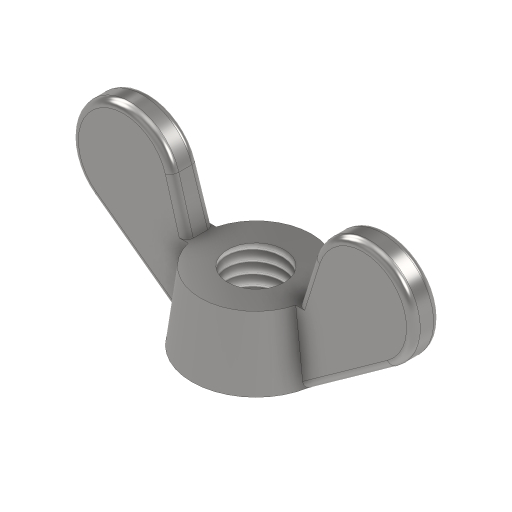
# Autodesk Inventor part: Part38FlyNut
Saved by Autodesk Inventor 2023.2 (Build 272271030, 271C)
## iProperties
Created: 2023-09-07
Part Number: Part38FlyNut
Material: Steel, Carbon
Document SubType Name: Modeling
Designer: User
Density: 7.85 g/cm^3
Appearance: Semi-Polished
Mass: 15.1733 g
Surface Area: 15.3566 cm^2
Volume: 1.9329 cm^3
Author: User
Autodesk Inventor part; units mm, degrees
ref_plane "YZ Plane" through (0, 0, 0) normal (1, 0, 0) x (0, 1, 0)
ref_plane "XZ Plane" through (0, 0, 0) normal (0, 1, 0) x (-1, 0, 0)
ref_plane "XY Plane" through (0, 0, 0) normal (0, 0, 1) x (1, 0, 0)
sketch "Sketch1" plane through (0, 0, 0) normal (1, 0, 0) x (0, 1, 0)
  line L0 (0, 1.75) -> (18, 1.5)
  line L1 (18, 1.5) -> (18, -1.5)
  line L2 (18, -1.5) -> (0, -1.75)
  line L3 (0, -1.75) -> (0, 1.75)
  point P0 (0, 0)
  point P1 (0, 0)
  point P2 (18, 0)
  dimension "d0" = 3.5
  dimension "d1" = 3
  dimension "d2" = 18
  constraints: 8 end point, 2 midpoint, 1 coincident, 1 horizontal alignment, 1 parallel, 1 vertical
  measures "d0" distance of L2.end L0.start
  measures "d1" distance of L0.end L1.end
  measures "d2" distance between parallel lines of L3 L1
extrude "Extrusion1" add sketch "Sketch1" along normal mid plane 40
sketch "Sketch2" plane through (0, 0, 0) normal (0, 0, 1) x (1, 0, 0)
  line L0 (-6.5, 8) -> (6.5, 8)
  line L1 (6.5, 8) -> (7.5, 0)
  line L2 (7.5, 0) -> (-7.5, 0)
  line L3 (-7.5, 0) -> (-6.5, 8)
  arc A0 (17.4822, 7.1138) -> (8.263, 13.7569) centre (14, 12) ccw
  line L4 (-20, 18) -> (20, 18) projected
  line L5 (20, 0) -> (20, 18) projected
  line L6 (8.263, 13.7569) -> (6.5, 8)
  line L7 (17.4822, 7.1138) -> (7.5, 0)
  line L8 (0, -4.0751) -> (0, 24.4507) projected
  arc A1 (-8.263, 13.7569) -> (-17.4822, 7.1138) centre (-14, 12) ccw
  line L9 (-8.263, 13.7569) -> (-6.5, 8)
  line L10 (-17.4822, 7.1138) -> (-7.5, 0)
  point P0 (0, 0)
  point P1 (0, 0)
  dimension "d5" = 8
  dimension "d6" = 15
  dimension "d7" = 13
  dimension "d8" = 6
  constraints: 16 end point, 4 point on circle, 4 tangent, 3 symmetric about line, 2 centre point, 1 coincident, 1 equal length, 1 horizontal, 1 midpoint, 1 parallel, 1 other
  measures "d5" distance between parallel lines of L2 L0
  measures "d6" distance of L1.end L2.end
  measures "d7" distance of L0.start L0.end
  measures "d8" radius of A0
extrude "Extrusion2" cut sketch "Sketch2" along normal mid plane 3.5 contours L0 L8 L2 L3 | L3 L10 A1 L9 | L0 L1 L2 L8 | L6 A0 L7 L1 keep common part
sketch "Sketch3" plane through (0, 0, 0) normal (0, 0, 1) x (1, 0, 0)
  line L0 (6.5, 8) -> (7.5, 0) projected
  line L1 (0, -4.0751) -> (0, 24.4507) projected
  line L2 (0, 8) -> (6.5, 8)
  line L3 (0, 0) -> (7.5, 0)
  constraints: 4 end point, 1 horizontal, 1 perpendicular, 1 point on line
revolve "Revolution1" add sketch "Sketch3" angle 360 about axis through (0, -4.0751, 0) along (0, 1, 0)
sketch "Sketch5" plane through (6.5, 8, 1.6389) normal (0, 1, 0) x (1, 0, 0)
  arc A0 (-0.21, 3.2778) -> (-12.79, 3.2778) centre (-6.5, 1.6389) ccw projected
  point P0 (-6.5, 1.6389)
  constraints: 1 coincident
hole "Hole1" at (0, 8, 0) direction (0, -1, 0) diameter 6.647 end through all thread size "M8x1.25" class "6H" standard "ISO Metric profile"
fillet "Fillet1" radius 0.8 16 edges at (-10.4322, 16.824, 1.5163) (-19.3335, 9.2516, 1.6215) (-7.3815, 10.8784, 1.5989) (-12.4911, 3.5569, 1.7006) (-12.4911, 3.5569, -1.7006) (-7.3815, 10.8784, -1.5989) (-19.3335, 9.2516, -1.6215) (-10.4322, 16.824, -1.5163) (7.3815, 10.8784, -1.5989) (12.4911, 3.5569, -1.7006) (10.4322, 16.824, -1.5163) (19.3335, 9.2516, -1.6215) (12.4911, 3.5569, 1.7006) (7.3815, 10.8784, 1.5989) (19.3335, 9.2516, 1.6215) (10.4322, 16.824, 1.5163)
chamfer "Chamfer1" distance 0.6765 angle 30 1 edges at (0, 0, -3.3235) measured on face at (-6.0998, 0, -0.1335)
equation "\"d9\" = d0"
body "Solid1"
